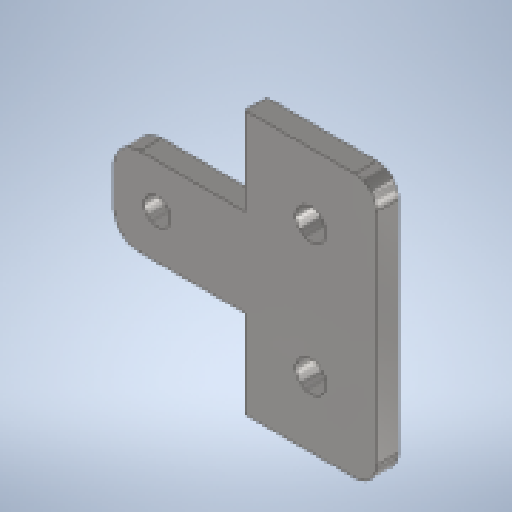
# Autodesk Inventor part: HCMUTE-CDT23-BAT_CANG_BANG_TAI
Saved by Autodesk Inventor 2023 (Build 270158000, 158)
## iProperties
Created: 2023-11-19
Part Number: HCMUTE-CDT23-BAT_CANG_BANG_TAI
Material: Stainless Steel
Document SubType Name: Sheet Metal
Designer: havie
Density: 8 g/cm^3
Sheet Metal Rule: Default_mm
Appearance: Semi-Polished
Author: havie
Autodesk Inventor part; units mm, degrees
ref_plane "YZ Plane" through (0, 0, 0) normal (1, 0, 0) x (0, 1, 0)
ref_plane "XZ Plane" through (0, 0, 0) normal (0, 1, 0) x (-1, 0, 0)
ref_plane "XY Plane" through (0, 0, 0) normal (0, 0, 1) x (1, 0, 0)
sketch "Sketch1" plane through (0, 0, 0) normal (1, 0, 0) x (0, 1, 0)
  line L0 (-25, 30) -> (25, 30)
  line L1 (30, 25) -> (30, -25)
  line L2 (25, -30) -> (-25, -30)
  line L3 (-30, -25) -> (-30, 25)
  line L4 (-30, 30) -> (30, -30) construction
  line L5 (30, 30) -> (-30, -30) construction
  arc A0 (-25, 30) -> (-30, 25) centre (-25, 25) ccw
  arc A1 (-30, -25) -> (-25, -30) centre (-25, -25) ccw
  arc A2 (25, -30) -> (30, -25) centre (25, -25) ccw
  arc A3 (30, 25) -> (25, 30) centre (25, 25) ccw
  circle A4 centre (-20, 0) radius 4
  circle A5 centre (15, 15) radius 3.5
  circle A6 centre (15, -15) radius 3.5
  point P0 (0, 0)
  dimension "d0" = 60
  dimension "d1" = 60
  dimension "d6" = 5
  dimension "d7" = 8
  dimension "d10" = 15
  dimension "d11" = 30
  dimension "d12" = 15
  dimension "d13" = 7
  dimension "d14" = 35
  measures "d0" distance of L4.end L5.end
  measures "d1" distance of L5.end L4.start
  measures "d6" radius of A0
  measures "d7" diameter of A4
  measures "d10" distance from line of L2 A6.centre
  measures "d11" distance of A5.centre A6.centre
  measures "d12" distance from line of L1 A5.centre
  measures "d13" diameter of A5
  measures "d14" horizontal distance of A5.centre A4.centre
extrude "Plate1" add sketch "Sketch1" along normal mid plane 5
sketch "Sketch2" plane through (2.5, 0, 0) normal (1, 0, 0) x (0, 0, -1)
  line L0 (-30, -30) -> (-10, -30)
  line L1 (-10, -30) -> (-10, 0)
  line L2 (-10, 0) -> (-30, 0)
  line L3 (-30, 0) -> (-30, -30)
  line L4 (30, -30) -> (10, -30)
  line L5 (10, -30) -> (10, 0)
  line L6 (10, 0) -> (30, 0)
  line L7 (30, 0) -> (30, -30)
  circle A0 centre (-15, 15) radius 3.5 projected
  circle A1 centre (0, -20) radius 4 projected
  line L8 (-30, -25) -> (-30, 25) construction
  point P0 (0, 0)
  dimension "d15" = 15
  dimension "d17" = 10
  dimension "d18" = 10
  dimension "d19" = 30
  constraints: 16 end point, 4 parallel, 2 horizontal, 2 perpendicular, 2 point on line, 1 collinear, 1 midpoint
  measures "d15" distance from line of A0.centre L2
  measures "d17" distance from line of A1.centre L1
  measures "d18" distance from line of A1.centre L5
  measures "d19" distance of L2.end L0.start
extrude "Cut1" cut sketch "Sketch2" against normal blind 5 contours L3 L2 L1 L0 | L4 L5 L6 L7
fillet "Corner Round1" radius 6 2 edges at (0, -30, 10) (0, -30, -10)
equation "\"d20\" = Thickness"
equation "\"d9\" = Thickness"
equation "\"BendRadius\" = Thickness"
equation "\"BendReliefWidth\" = Thickness"
equation "\"BendReliefDepth\" = 0.5 * Thickness"
equation "\"TransitionRadius\" = BendRadius"
equation "\"JacobiRadiusSize\" = BendRadius"
equation "\"GapSize\" = Thickness"
equation "\"Thickness\" = 5"
body "Solid1"
